Autodesk Fusion 360 part; units mm, degrees
note: some values were not read from the file. Set by a fixed rule: which sketch regions a step uses; which face or edge a step refers to.
(part 2 of 2)
sketch "Sketch17" plane through (0, 0, 1) normal (0, 0, 1) x (-1, 0, 0)
  line L0 (9.737, -2.175) -> (9.3184, -3.325)
  line L1 (9.3184, -3.325) -> (9.1145, -3.325)
  line L2 (9.1145, -3.325) -> (8.6959, -2.175)
  line L3 (8.6959, -2.175) -> (8.8596, -2.175)
  line L4 (8.8596, -2.175) -> (9.2203, -3.1868)
  line L5 (9.2203, -3.1868) -> (9.581, -2.175)
  line L6 (9.581, -2.175) -> (9.737, -2.175)
  spline S0 degree 3 poles (10.7997, -3.2416) (10.7862, -3.2475) (10.7604, -3.2588) (10.735, -3.2707) (10.7229, -3.2763) knots 0 0 0 0 0.004426 0.008434 0.008434 0.008434 0.008434
  spline S1 degree 3 poles (10.7229, -3.2763) (10.7097, -3.2821) (10.6803, -3.2949) (10.6498, -3.3048) (10.6329, -3.3103) knots 0 0 0 0 0.004301 0.009623 0.009623 0.009623 0.009623
  spline S2 degree 3 poles (10.6329, -3.3103) (10.6166, -3.3151) (10.5828, -3.3249) (10.5483, -3.3319) (10.5305, -3.3354) knots 0 0 0 0 0.005099 0.010541 0.010541 0.010541 0.010541
  spline S3 degree 3 poles (10.5305, -3.3354) (10.5112, -3.3385) (10.4709, -3.3448) (10.4302, -3.3455) (10.4089, -3.3459) knots 0 0 0 0 0.005855 0.012222 0.012222 0.012222 0.012222
  spline S4 degree 3 poles (10.4089, -3.3459) (10.3688, -3.3446) (10.2915, -3.3422) (10.2172, -3.321) (10.1814, -3.3107) knots 0 0 0 0 0.011974 0.023094 0.023094 0.023094 0.023094
  spline S5 degree 3 poles (10.1814, -3.3107) (10.1485, -3.2974) (10.0829, -3.2709) (10.0298, -3.224) (10.0034, -3.2007) knots 0 0 0 0 0.010576 0.021066 0.021066 0.021066 0.021066
  spline S6 degree 3 poles (10.0034, -3.2007) (9.9798, -3.1739) (9.9308, -3.1182) (9.9023, -3.0497) (9.8876, -3.0141) knots 0 0 0 0 0.010631 0.022091 0.022091 0.022091 0.022091
  spline S7 degree 3 poles (9.8876, -3.0141) (9.8754, -2.9736) (9.8497, -2.8879) (9.8472, -2.7984) (9.8459, -2.7512) knots 0 0 0 0 0.012625 0.02673 0.02673 0.02673 0.02673
  spline S8 degree 3 poles (9.8459, -2.7512) (9.8472, -2.706) (9.8498, -2.6195) (9.8743, -2.5366) (9.886, -2.4971) knots 0 0 0 0 0.013495 0.025821 0.025821 0.025821 0.025821
  spline S9 degree 3 poles (9.886, -2.4971) (9.9006, -2.4615) (9.929, -2.3921) (9.978, -2.3355) (10.0019, -2.3078) knots 0 0 0 0 0.011435 0.022319 0.022319 0.022319 0.022319
  spline S10 degree 3 poles (10.0019, -2.3078) (10.0279, -2.2843) (10.0806, -2.2364) (10.146, -2.208) (10.1791, -2.1935) knots 0 0 0 0 0.01045 0.021218 0.021218 0.021218 0.021218
  spline S11 degree 3 poles (10.1791, -2.1935) (10.2154, -2.1821) (10.2904, -2.1583) (10.369, -2.1556) (10.4097, -2.1541) knots 0 0 0 0 0.011349 0.023485 0.023485 0.023485 0.023485
  spline S12 degree 3 poles (10.4097, -2.1541) (10.4406, -2.1551) (10.503, -2.157) (10.564, -2.17) (10.5946, -2.1765) knots 0 0 0 0 0.009275 0.018666 0.018666 0.018666 0.018666
  spline S13 degree 3 poles (10.5946, -2.1765) (10.6274, -2.186) (10.698, -2.2064) (10.7642, -2.2383) (10.7997, -2.2553) knots 0 0 0 0 0.010219 0.022001 0.022001 0.022001 0.022001
  line L7 (10.7997, -2.2553) -> (10.7997, -2.4368)
  line L8 (10.7997, -2.4368) -> (10.7881, -2.4368)
  spline S14 degree 3 poles (10.7881, -2.4368) (10.7574, -2.4125) (10.6992, -2.3663) (10.6316, -2.3355) (10.5997, -2.321) knots 0 0 0 0 0.011694 0.022195 0.022195 0.022195 0.022195
  spline S15 degree 3 poles (10.5997, -2.321) (10.5677, -2.3104) (10.5027, -2.2889) (10.4344, -2.2861) (10.3996, -2.2847) knots 0 0 0 0 0.010049 0.020419 0.020419 0.020419 0.020419
  spline S16 degree 3 poles (10.3996, -2.2847) (10.3717, -2.2857) (10.318, -2.2876) (10.267, -2.3046) (10.2425, -2.3129) knots 0 0 0 0 0.008323 0.016042 0.016042 0.016042 0.016042
  spline S17 degree 3 poles (10.2425, -2.3129) (10.2196, -2.3237) (10.1731, -2.3459) (10.1364, -2.3821) (10.1177, -2.4005) knots 0 0 0 0 0.00753 0.015341 0.015341 0.015341 0.015341
  spline S18 degree 3 poles (10.1177, -2.4005) (10.1008, -2.4217) (10.0652, -2.466) (10.0452, -2.5191) (10.0347, -2.5469) knots 0 0 0 0 0.008089 0.01692 0.01692 0.01692 0.01692
  spline S19 degree 3 poles (10.0347, -2.5469) (10.026, -2.5785) (10.0077, -2.6453) (10.0059, -2.7146) (10.005, -2.7512) knots 0 0 0 0 0.009786 0.020711 0.020711 0.020711 0.020711
  spline S20 degree 3 poles (10.005, -2.7512) (10.0059, -2.789) (10.0077, -2.86) (10.0282, -2.928) (10.0378, -2.9597) knots 0 0 0 0 0.011306 0.021194 0.021194 0.021194 0.021194
  spline S21 degree 3 poles (10.0378, -2.9597) (10.049, -2.9869) (10.0703, -3.0384) (10.1056, -3.0814) (10.1224, -3.1018) knots 0 0 0 0 0.008762 0.016619 0.016619 0.016619 0.016619
  spline S22 degree 3 poles (10.1224, -3.1018) (10.1411, -3.1196) (10.1783, -3.155) (10.2253, -3.1759) (10.2486, -3.1864) knots 0 0 0 0 0.007685 0.015297 0.015297 0.015297 0.015297
  spline S23 degree 3 poles (10.2486, -3.1864) (10.2732, -3.1944) (10.3228, -3.2105) (10.3749, -3.2127) (10.4012, -3.2138) knots 0 0 0 0 0.007704 0.015563 0.015563 0.015563 0.015563
  spline S24 degree 3 poles (10.4012, -3.2138) (10.4371, -3.2123) (10.5079, -3.2094) (10.5751, -3.187) (10.6082, -3.1759) knots 0 0 0 0 0.010739 0.021135 0.021135 0.021135 0.021135
  spline S25 degree 3 poles (10.6082, -3.1759) (10.6401, -3.1615) (10.7055, -3.1319) (10.7607, -3.0859) (10.7889, -3.0624) knots 0 0 0 0 0.010474 0.02143 0.02143 0.02143 0.02143
  line L9 (10.7889, -3.0624) -> (10.7997, -3.0624)
  line L10 (10.7997, -3.0624) -> (10.7997, -3.2416)
  spline S26 degree 3 poles (11.9361, 2.3894) (11.9335, 2.3388) (11.9284, 2.2398) (11.8876, 2.1494) (11.8677, 2.1052) knots 0 0 0 0 0.015042 0.029461 0.029461 0.029461 0.029461
  spline S27 degree 3 poles (11.8677, 2.1052) (11.8435, 2.0653) (11.7959, 1.9873) (11.722, 1.9337) (11.6858, 1.9075) knots 0 0 0 0 0.013837 0.027105 0.027105 0.027105 0.027105
  spline S28 degree 3 poles (11.6858, 1.9075) (11.6585, 1.8923) (11.603, 1.8614) (11.5414, 1.8454) (11.5101, 1.8372) knots 0 0 0 0 0.009326 0.018991 0.018991 0.018991 0.018991
  spline S29 degree 3 poles (11.5101, 1.8372) (11.4728, 1.8309) (11.3883, 1.8167) (11.3027, 1.816) (11.2549, 1.8156) knots 0 0 0 0 0.011344 0.025652 0.025652 0.025652 0.025652
  line L11 (11.2549, 1.8156) -> (10.9645, 1.8156)
  line L12 (10.9645, 1.8156) -> (10.9645, 2.9656)
  line L13 (10.9645, 2.9656) -> (11.2518, 2.9656)
  spline S30 degree 3 poles (11.2518, 2.9656) (11.3023, 2.9651) (11.3922, 2.9644) (11.4806, 2.9483) (11.5194, 2.9412) knots 0 0 0 0 0.015121 0.026915 0.026915 0.026915 0.026915
  spline S31 degree 3 poles (11.5194, 2.9412) (11.5504, 2.9328) (11.609, 2.917) (11.6623, 2.888) (11.6874, 2.8744) knots 0 0 0 0 0.009606 0.018133 0.018133 0.018133 0.018133
  spline S32 degree 3 poles (11.6874, 2.8744) (11.7244, 2.8479) (11.7983, 2.7949) (11.8464, 2.7177) (11.8704, 2.679) knots 0 0 0 0 0.013501 0.027009 0.027009 0.027009 0.027009
  spline S33 degree 3 poles (11.8704, 2.679) (11.8895, 2.6352) (11.9298, 2.5429) (11.9339, 2.4422) (11.9361, 2.3894) knots 0 0 0 0 0.014221 0.029928 0.029928 0.029928 0.029928
  line L14 (10.3066, 0.4767) -> (9.7528, -0.9598)
  line L15 (9.7528, -0.9598) -> (9.6192, -0.9598)
  line L16 (9.6192, -0.9598) -> (10.1706, 0.4767)
  line L17 (10.1706, 0.4767) -> (10.3066, 0.4767)
  line L18 (9.5366, -0.725) -> (9.0824, -0.725)
  line L19 (9.0824, -0.725) -> (9.0824, -0.6076)
  line L20 (9.0824, -0.6076) -> (9.233, -0.6076)
  line L21 (9.233, -0.6076) -> (9.233, 0.3076)
  line L22 (9.233, 0.3076) -> (9.0824, 0.3076)
  line L23 (9.0824, 0.3076) -> (9.0824, 0.425)
  line L24 (9.0824, 0.425) -> (9.5366, 0.425)
  line L25 (9.5366, 0.425) -> (9.5366, 0.3076)
  line L26 (9.5366, 0.3076) -> (9.3859, 0.3076)
  line L27 (9.3859, 0.3076) -> (9.3859, -0.6076)
  line L28 (9.3859, -0.6076) -> (9.5366, -0.6076)
  line L29 (9.5366, -0.6076) -> (9.5366, -0.725)
  spline S34 degree 3 poles (11.9041, -3.2416) (11.8906, -3.2475) (11.8649, -3.2588) (11.8394, -3.2707) (11.8273, -3.2763) knots 0 0 0 0 0.004426 0.008434 0.008434 0.008434 0.008434
  spline S35 degree 3 poles (11.8273, -3.2763) (11.8141, -3.2821) (11.7847, -3.2949) (11.7542, -3.3048) (11.7373, -3.3103) knots 0 0 0 0 0.004301 0.009623 0.009623 0.009623 0.009623
  spline S36 degree 3 poles (11.7373, -3.3103) (11.721, -3.3151) (11.6872, -3.3249) (11.6528, -3.3319) (11.635, -3.3354) knots 0 0 0 0 0.005099 0.010541 0.010541 0.010541 0.010541
  spline S37 degree 3 poles (11.635, -3.3354) (11.6157, -3.3385) (11.5754, -3.3448) (11.5346, -3.3455) (11.5133, -3.3459) knots 0 0 0 0 0.005855 0.012222 0.012222 0.012222 0.012222
  spline S38 degree 3 poles (11.5133, -3.3459) (11.4733, -3.3446) (11.396, -3.3422) (11.3217, -3.321) (11.2859, -3.3107) knots 0 0 0 0 0.011974 0.023094 0.023094 0.023094 0.023094
  spline S39 degree 3 poles (11.2859, -3.3107) (11.2529, -3.2974) (11.1873, -3.2709) (11.1343, -3.224) (11.1079, -3.2007) knots 0 0 0 0 0.010576 0.021066 0.021066 0.021066 0.021066
  spline S40 degree 3 poles (11.1079, -3.2007) (11.0843, -3.1739) (11.0352, -3.1182) (11.0068, -3.0497) (10.992, -3.0141) knots 0 0 0 0 0.010631 0.022091 0.022091 0.022091 0.022091
  spline S41 degree 3 poles (10.992, -3.0141) (10.9799, -2.9736) (10.9541, -2.8879) (10.9516, -2.7984) (10.9503, -2.7512) knots 0 0 0 0 0.012625 0.02673 0.02673 0.02673 0.02673
  spline S42 degree 3 poles (10.9503, -2.7512) (10.9517, -2.706) (10.9542, -2.6195) (10.9788, -2.5366) (10.9905, -2.4971) knots 0 0 0 0 0.013495 0.025821 0.025821 0.025821 0.025821
  spline S43 degree 3 poles (10.9905, -2.4971) (11.005, -2.4615) (11.0334, -2.3921) (11.0824, -2.3355) (11.1063, -2.3078) knots 0 0 0 0 0.011435 0.022319 0.022319 0.022319 0.022319
  spline S44 degree 3 poles (11.1063, -2.3078) (11.1323, -2.2843) (11.185, -2.2364) (11.2504, -2.208) (11.2836, -2.1935) knots 0 0 0 0 0.01045 0.021218 0.021218 0.021218 0.021218
  spline S45 degree 3 poles (11.2836, -2.1935) (11.3198, -2.1821) (11.3948, -2.1583) (11.4735, -2.1556) (11.5141, -2.1541) knots 0 0 0 0 0.011349 0.023485 0.023485 0.023485 0.023485
  spline S46 degree 3 poles (11.5141, -2.1541) (11.5451, -2.1551) (11.6074, -2.157) (11.6684, -2.17) (11.6991, -2.1765) knots 0 0 0 0 0.009275 0.018666 0.018666 0.018666 0.018666
  spline S47 degree 3 poles (11.6991, -2.1765) (11.7319, -2.186) (11.8024, -2.2064) (11.8687, -2.2383) (11.9041, -2.2553) knots 0 0 0 0 0.010219 0.022001 0.022001 0.022001 0.022001
  line L30 (11.9041, -2.2553) -> (11.9041, -2.4368)
  line L31 (11.9041, -2.4368) -> (11.8925, -2.4368)
  spline S48 degree 3 poles (11.8925, -2.4368) (11.8619, -2.4125) (11.8037, -2.3663) (11.7361, -2.3355) (11.7041, -2.321) knots 0 0 0 0 0.011694 0.022195 0.022195 0.022195 0.022195
  spline S49 degree 3 poles (11.7041, -2.321) (11.6721, -2.3104) (11.6072, -2.2889) (11.5388, -2.2861) (11.5041, -2.2847) knots 0 0 0 0 0.010049 0.020419 0.020419 0.020419 0.020419
  spline S50 degree 3 poles (11.5041, -2.2847) (11.4762, -2.2857) (11.4224, -2.2876) (11.3714, -2.3046) (11.3469, -2.3129) knots 0 0 0 0 0.008323 0.016042 0.016042 0.016042 0.016042
  spline S51 degree 3 poles (11.3469, -2.3129) (11.3241, -2.3237) (11.2775, -2.3459) (11.2408, -2.3821) (11.2222, -2.4005) knots 0 0 0 0 0.00753 0.015341 0.015341 0.015341 0.015341
  spline S52 degree 3 poles (11.2222, -2.4005) (11.2052, -2.4217) (11.1697, -2.466) (11.1496, -2.5191) (11.1391, -2.5469) knots 0 0 0 0 0.008089 0.01692 0.01692 0.01692 0.01692
  spline S53 degree 3 poles (11.1391, -2.5469) (11.1305, -2.5785) (11.1121, -2.6453) (11.1103, -2.7146) (11.1094, -2.7512) knots 0 0 0 0 0.009786 0.020711 0.020711 0.020711 0.020711
  spline S54 degree 3 poles (11.1094, -2.7512) (11.1104, -2.789) (11.1122, -2.86) (11.1327, -2.928) (11.1422, -2.9597) knots 0 0 0 0 0.011306 0.021194 0.021194 0.021194 0.021194
  spline S55 degree 3 poles (11.1422, -2.9597) (11.1534, -2.9869) (11.1747, -3.0384) (11.2101, -3.0814) (11.2268, -3.1018) knots 0 0 0 0 0.008762 0.016619 0.016619 0.016619 0.016619
  spline S56 degree 3 poles (11.2268, -3.1018) (11.2455, -3.1196) (11.2828, -3.155) (11.3297, -3.1759) (11.3531, -3.1864) knots 0 0 0 0 0.007685 0.015297 0.015297 0.015297 0.015297
  spline S57 degree 3 poles (11.3531, -3.1864) (11.3776, -3.1944) (11.4272, -3.2105) (11.4793, -3.2127) (11.5056, -3.2138) knots 0 0 0 0 0.007704 0.015563 0.015563 0.015563 0.015563
  spline S58 degree 3 poles (11.5056, -3.2138) (11.5416, -3.2123) (11.6124, -3.2094) (11.6795, -3.187) (11.7126, -3.1759) knots 0 0 0 0 0.010739 0.021135 0.021135 0.021135 0.021135
  spline S59 degree 3 poles (11.7126, -3.1759) (11.7446, -3.1615) (11.81, -3.1319) (11.8651, -3.0859) (11.8933, -3.0624) knots 0 0 0 0 0.010474 0.02143 0.02143 0.02143 0.02143
  line L32 (11.8933, -3.0624) -> (11.9041, -3.0624)
  line L33 (11.9041, -3.0624) -> (11.9041, -3.2416)
  line L34 (15.2, 3.58) -> (15.2, 3.38)
  line L35 (15.2, 3.38) -> (15.2, 1.38)
  line L36 (15.2, 1.38) -> (15.2, -1.7)
  line L37 (15.2, -1.7) -> (15.2, -3.7)
  line L38 (15.2, -3.7) -> (15.2, -3.9)
  line L39 (15.2, -3.9) -> (13, -3.9)
  line L40 (13, -3.9) -> (12.8, -3.9)
  line L41 (12.8, -3.9) -> (12.8, -1.7)
  line L42 (12.8, -1.7) -> (12.8, 1.38)
  line L43 (12.8, 1.38) -> (12.8, 3.38)
  line L44 (12.8, 3.38) -> (12.8, 3.58)
  line L45 (12.8, 3.58) -> (15.2, 3.58)
  circle A0 centre (-9.5, 0) radius 6.3
  line L46 (6.875, 3.125) -> (6.375, 3.125)
  line L47 (6.375, 3.125) -> (6.375, 3.1251)
  line L48 (6.375, 3.1251) -> (5.375, 3.1251)
  line L49 (5.375, 3.1251) -> (5.375, 3.125)
  line L50 (5.375, 3.125) -> (4.875, 3.125)
  line L51 (4.875, 3.125) -> (4.875, 3.875)
  line L52 (4.875, 3.875) -> (5.375, 3.875)
  line L53 (5.375, 3.875) -> (5.375, 3.8749)
  line L54 (5.375, 3.8749) -> (6.375, 3.8749)
  line L55 (6.375, 3.8749) -> (6.375, 3.875)
  line L56 (6.375, 3.875) -> (6.875, 3.875)
  line L57 (6.875, 3.875) -> (6.875, 3.125)
  line L58 (-16, 6.5) -> (-16, -6.5)
  line L59 (-16, -6.5) -> (16, -6.5)
  line L60 (16, -6.5) -> (16, 6.5)
  line L61 (16, 6.5) -> (-16, 6.5)
  line L62 (4.55, 0.25) -> (4.7951, 0.25)
  line L63 (4.7951, 0.25) -> (5.25, 0.25)
  line L64 (5.25, 0.25) -> (5.25, 1.5)
  line L65 (5.25, 1.5) -> (6.5, 1.5)
  line L66 (6.5, 1.5) -> (6.5, 1.4)
  line L67 (6.5, 1.4) -> (6.9549, 1.4)
  line L68 (6.9549, 1.4) -> (7.2, 1.4)
  arc A1 (7.3, 1.3) -> (7.2, 1.4) centre (7.2, 1.3) ccw
  line L69 (7.3, 1.3) -> (7.3, 1)
  arc A2 (7.2, 0.9) -> (7.3, 1) centre (7.2, 1) ccw
  line L70 (7.2, 0.9) -> (6.9549, 0.9)
  line L71 (6.9549, 0.9) -> (6.5, 0.9)
  line L72 (6.5, 0.9) -> (6.5, -0.9)
  line L73 (6.5, -0.9) -> (6.9549, -0.9)
  line L74 (6.9549, -0.9) -> (7.2, -0.9)
  arc A3 (7.3, -1) -> (7.2, -0.9) centre (7.2, -1) ccw
  line L75 (7.3, -1) -> (7.3, -1.3)
  arc A4 (7.2, -1.4) -> (7.3, -1.3) centre (7.2, -1.3) ccw
  line L76 (7.2, -1.4) -> (6.9549, -1.4)
  line L77 (6.9549, -1.4) -> (6.5, -1.4)
  line L78 (6.5, -1.4) -> (6.5, -1.5)
  line L79 (6.5, -1.5) -> (5.25, -1.5)
  line L80 (5.25, -1.5) -> (5.25, -0.25)
  line L81 (5.25, -0.25) -> (4.7951, -0.25)
  line L82 (4.7951, -0.25) -> (4.55, -0.25)
  arc A5 (4.45, -0.15) -> (4.55, -0.25) centre (4.55, -0.15) ccw
  line L83 (4.45, -0.15) -> (4.45, 0.15)
  arc A6 (4.55, 0.25) -> (4.45, 0.15) centre (4.55, 0.15) ccw
  circle A7 centre (0.5, 0) radius 2.25
  line L84 (10.6586, 1.8156) -> (10.4694, 1.8156)
  line L85 (10.4694, 1.8156) -> (9.9241, 2.8443)
  line L86 (9.9241, 2.8443) -> (9.9241, 1.8156)
  line L87 (9.9241, 1.8156) -> (9.7813, 1.8156)
  line L88 (9.7813, 1.8156) -> (9.7813, 2.9656)
  line L89 (9.7813, 2.9656) -> (10.0184, 2.9656)
  line L90 (10.0184, 2.9656) -> (10.5157, 2.0264)
  line L91 (10.5157, 2.0264) -> (10.5157, 2.9656)
  line L92 (10.5157, 2.9656) -> (10.6586, 2.9656)
  line L93 (10.6586, 2.9656) -> (10.6586, 1.8156)
  spline S60 degree 3 poles (9.514, 1.9005) (9.4814, 1.8864) (9.4142, 1.8574) (9.3442, 1.8361) (9.3082, 1.8252) knots 0 0 0 0 0.010655 0.021932 0.021932 0.021932 0.021932
  spline S61 degree 3 poles (9.3082, 1.8252) (9.2718, 1.8159) (9.201, 1.7977) (9.1279, 1.7946) (9.0923, 1.7932) knots 0 0 0 0 0.011237 0.021877 0.021877 0.021877 0.021877
  spline S62 degree 3 poles (9.0923, 1.7932) (9.0491, 1.7945) (8.9655, 1.7971) (8.8849, 1.8194) (8.846, 1.8302) knots 0 0 0 0 0.012912 0.024995 0.024995 0.024995 0.024995
  spline S63 degree 3 poles (8.846, 1.8302) (8.8103, 1.8438) (8.7406, 1.8705) (8.6832, 1.9181) (8.6552, 1.9414) knots 0 0 0 0 0.011357 0.022216 0.022216 0.022216 0.022216
  spline S64 degree 3 poles (8.6552, 1.9414) (8.63, 1.9684) (8.5784, 2.0238) (8.548, 2.0932) (8.5324, 2.1287) knots 0 0 0 0 0.010986 0.02254 0.02254 0.02254 0.02254
  spline S65 degree 3 poles (8.5324, 2.1287) (8.5198, 2.1691) (8.4931, 2.2546) (8.4905, 2.3443) (8.4892, 2.3917) knots 0 0 0 0 0.012617 0.026763 0.026763 0.026763 0.026763
  spline S66 degree 3 poles (8.4892, 2.3917) (8.4943, 2.4771) (8.5039, 2.639) (8.6033, 2.7666) (8.6502, 2.8269) knots 0 0 0 0 0.024993 0.047384 0.047384 0.047384 0.047384
  spline S67 degree 3 poles (8.6502, 2.8269) (8.7114, 2.8734) (8.8417, 2.9723) (9.0055, 2.9815) (9.0923, 2.9864) knots 0 0 0 0 0.022541 0.047966 0.047966 0.047966 0.047966
  spline S68 degree 3 poles (9.0923, 2.9864) (9.1255, 2.9854) (9.193, 2.9832) (9.2591, 2.9697) (9.2928, 2.9628) knots 0 0 0 0 0.009932 0.020212 0.020212 0.020212 0.020212
  spline S69 degree 3 poles (9.2928, 2.9628) (9.3285, 2.9532) (9.4042, 2.9326) (9.4756, 2.9001) (9.5133, 2.8829) knots 0 0 0 0 0.011094 0.023489 0.023489 0.023489 0.023489
  line L94 (9.5133, 2.8829) -> (9.5133, 2.7014)
  line L95 (9.5133, 2.7014) -> (9.4994, 2.7014)
  spline S70 degree 3 poles (9.4994, 2.7014) (9.4896, 2.7086) (9.4669, 2.7255) (9.4433, 2.7411) (9.4299, 2.7501) knots 0 0 0 0 0.003634 0.008486 0.008486 0.008486 0.008486
  spline S71 degree 3 poles (9.4299, 2.7501) (9.415, 2.7596) (9.3861, 2.778) (9.3552, 2.793) (9.3403, 2.8003) knots 0 0 0 0 0.005295 0.010277 0.010277 0.010277 0.010277
  spline S72 degree 3 poles (9.3403, 2.8003) (9.3215, 2.808) (9.2821, 2.8242) (9.2409, 2.8346) (9.2194, 2.84) knots 0 0 0 0 0.006094 0.012739 0.012739 0.012739 0.012739
  spline S73 degree 3 poles (9.2194, 2.84) (9.1954, 2.8447) (9.1448, 2.8544) (9.0932, 2.8554) (9.0661, 2.8559) knots 0 0 0 0 0.007309 0.015438 0.015438 0.015438 0.015438
  spline S74 degree 3 poles (9.0661, 2.8559) (9.0059, 2.8516) (8.8903, 2.8434) (8.8027, 2.7681) (8.7606, 2.7319) knots 0 0 0 0 0.017566 0.033757 0.033757 0.033757 0.033757
  spline S75 degree 3 poles (8.7606, 2.7319) (8.7279, 2.6849) (8.6579, 2.5844) (8.6516, 2.4617) (8.6483, 2.3963) knots 0 0 0 0 0.016847 0.036024 0.036024 0.036024 0.036024
  spline S76 degree 3 poles (8.6483, 2.3963) (8.6515, 2.3279) (8.6576, 2.2005) (8.7315, 2.0971) (8.7656, 2.0492) knots 0 0 0 0 0.020055 0.037342 0.037342 0.037342 0.037342
  spline S77 degree 3 poles (8.7656, 2.0492) (8.8098, 2.013) (8.9026, 1.9371) (9.0225, 1.9293) (9.0854, 1.9252) knots 0 0 0 0 0.016692 0.035066 0.035066 0.035066 0.035066
  spline S78 degree 3 poles (9.0854, 1.9252) (9.1101, 1.9258) (9.1598, 1.9271) (9.2087, 1.9356) (9.2333, 1.9399) knots 0 0 0 0 0.007414 0.014881 0.014881 0.014881 0.014881
  spline S79 degree 3 poles (9.2333, 1.9399) (9.2565, 1.9449) (9.3006, 1.9544) (9.3427, 1.9703) (9.3627, 1.9777) knots 0 0 0 0 0.007123 0.013495 0.013495 0.013495 0.013495
  line L96 (9.3627, 1.9777) -> (9.3627, 2.2596)
  line L97 (9.3627, 2.2596) -> (9.0545, 2.2596)
  line L98 (9.0545, 2.2596) -> (9.0545, 2.394)
  line L99 (9.0545, 2.394) -> (9.514, 2.394)
  line L100 (9.514, 2.394) -> (9.514, 1.9005)
  spline S80 degree 3 poles (11.3724, 0.2929) (11.3946, 0.2652) (11.4406, 0.2079) (11.4667, 0.1392) (11.4801, 0.1037) knots 0 0 0 0 0.0106 0.021894 0.021894 0.021894 0.021894
  spline S81 degree 3 poles (11.4801, 0.1037) (11.491, 0.0641) (11.514, -0.019) (11.5163, -0.1052) (11.5176, -0.1504) knots 0 0 0 0 0.012278 0.025768 0.025768 0.025768 0.025768
  spline S82 degree 3 poles (11.5176, -0.1504) (11.5163, -0.1956) (11.5139, -0.282) (11.4905, -0.3652) (11.4793, -0.4049) knots 0 0 0 0 0.013501 0.02582 0.02582 0.02582 0.02582
  spline S83 degree 3 poles (11.4793, -0.4049) (11.4658, -0.4402) (11.4398, -0.5082) (11.3943, -0.5649) (11.3724, -0.5922) knots 0 0 0 0 0.011276 0.021686 0.021686 0.021686 0.021686
  spline S84 degree 3 poles (11.3724, -0.5922) (11.3477, -0.6165) (11.2983, -0.6652) (11.2357, -0.6948) (11.2044, -0.7096) knots 0 0 0 0 0.010335 0.020625 0.020625 0.020625 0.020625
  spline S85 degree 3 poles (11.2044, -0.7096) (11.1701, -0.721) (11.0983, -0.7451) (11.0226, -0.7476) (10.9831, -0.7489) knots 0 0 0 0 0.01079 0.022581 0.022581 0.022581 0.022581
  spline S86 degree 3 poles (10.9831, -0.7489) (10.9442, -0.7475) (10.8687, -0.7447) (10.7972, -0.7205) (10.7626, -0.7088) knots 0 0 0 0 0.011619 0.022518 0.022518 0.022518 0.022518
  spline S87 degree 3 poles (10.7626, -0.7088) (10.7309, -0.694) (10.668, -0.6647) (10.6184, -0.6162) (10.5939, -0.5922) knots 0 0 0 0 0.010418 0.020646 0.020646 0.020646 0.020646
  spline S88 degree 3 poles (10.5939, -0.5922) (10.5718, -0.5647) (10.5263, -0.5078) (10.5003, -0.4397) (10.4869, -0.4045) knots 0 0 0 0 0.010503 0.021719 0.021719 0.021719 0.021719
  spline S89 degree 3 poles (10.4869, -0.4045) (10.476, -0.365) (10.453, -0.2819) (10.4507, -0.1957) (10.4494, -0.1504) knots 0 0 0 0 0.01224 0.025769 0.025769 0.025769 0.025769
  spline S90 degree 3 poles (10.4494, -0.1504) (10.4507, -0.1057) (10.4531, -0.0201) (10.4757, 0.0624) (10.4865, 0.1018) knots 0 0 0 0 0.013365 0.02557 0.02557 0.02557 0.02557
  spline S91 degree 3 poles (10.4865, 0.1018) (10.5, 0.1373) (10.5262, 0.2066) (10.5722, 0.2646) (10.5946, 0.2929) knots 0 0 0 0 0.011317 0.022078 0.022078 0.022078 0.022078
  spline S92 degree 3 poles (10.5946, 0.2929) (10.6189, 0.3168) (10.6684, 0.3653) (10.7314, 0.3941) (10.7634, 0.4088) knots 0 0 0 0 0.010132 0.020609 0.020609 0.020609 0.020609
  spline S93 degree 3 poles (10.7634, 0.4088) (10.7982, 0.4205) (10.8695, 0.4445) (10.9447, 0.4474) (10.9831, 0.4489) knots 0 0 0 0 0.010955 0.022439 0.022439 0.022439 0.022439
  spline S94 degree 3 poles (10.9831, 0.4489) (11.0226, 0.4475) (11.0986, 0.4448) (11.1706, 0.4202) (11.2052, 0.4084) knots 0 0 0 0 0.011773 0.022681 0.022681 0.022681 0.022681
  spline S95 degree 3 poles (11.2052, 0.4084) (11.2366, 0.3936) (11.2988, 0.3644) (11.348, 0.3166) (11.3724, 0.2929) knots 0 0 0 0 0.010345 0.020445 0.020445 0.020445 0.020445
  line L101 (4.875, 3.875) -> (6.875, 3.875)
  line L102 (6.875, 3.875) -> (6.875, 3.125)
  line L103 (6.875, 3.125) -> (4.875, 3.125)
  line L104 (4.875, 3.125) -> (4.875, 3.875)
  line L105 (5.25, 1.5) -> (6.5, 1.5)
  line L106 (6.5, 1.5) -> (6.5, -1.5)
  line L107 (6.5, -1.5) -> (5.25, -1.5)
  line L108 (5.25, -1.5) -> (5.25, 1.5)
  line L109 (7.075, 2.925) -> (4.675, 2.925)
  line L110 (4.675, 2.925) -> (4.675, 4.075)
  line L111 (4.675, 4.075) -> (7.075, 4.075)
  line L112 (7.075, 4.075) -> (7.075, 2.925)
  line L113 (7.375, 2.625) -> (4.375, 2.625)
  line L114 (4.375, 2.625) -> (4.375, 4.375)
  line L115 (4.375, 4.375) -> (7.375, 4.375)
  line L116 (7.375, 4.375) -> (7.375, 2.625)
  line L117 (6.7, -1.7) -> (5.05, -1.7)
  line L118 (5.05, -1.7) -> (5.05, 1.7)
  line L119 (5.05, 1.7) -> (6.7, 1.7)
  line L120 (6.7, 1.7) -> (6.7, -1.7)
  line L121 (7, -2) -> (4.75, -2)
  line L122 (4.75, -2) -> (4.75, 2)
  line L123 (4.75, 2) -> (7, 2)
  line L124 (7, 2) -> (7, -2)
  dimension "d293" = -0.2
  dimension "d294" = -0.5
  dimension "d295" = -0.2
  dimension "d296" = -0.5
  constraint horizontal L101
  constraint vertical L102
  constraint horizontal L103
  constraint vertical L104
  constraint coincident L46.start L57.end
  constraint coincident L51.end L52.start
  constraint horizontal L105
  constraint vertical L106
  constraint horizontal L107
  constraint vertical L108
  constraint coincident L78.end L79.start
  constraint coincident L64.end L65.start
extrude "Extrude33" add sketch "Sketch17" along normal blind 0.001 contours L62 L63 L67 L68 L118 L119 L120 L122 L123 L124 | L76 L77 L81 L82 L117 L118 L120 L121 L122 L124 | L70 L71 L73 L74 L120 L124 | L113 L114 L115 L116
equation "d95 = d94"
equation "d98 = d95"
equation "d99 = d98"
equation "d165 = d161"
equation "d166 = d160"
equation "d247 = d246"
named bodies: "Active"
